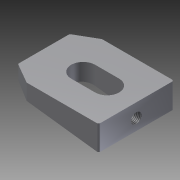
# Autodesk Inventor part: Wedge
Saved by Autodesk Inventor 2015 (Build 190159000, 159)
## iProperties
Shininess: 64.0
Angle Display Precision: 2
Document Length Units: 11272
Document Angle Units: 11279
Document Time Units: 11290
Document Mass Units: 11286
Document Length Units Precision: 3
Document Angle Units Precision: 2
Created: 2004-03-19
Part Number: Wedge
Document SubType Name: Modeling
Designer: bhandley
Material: Generic
Density: 1 g/cm^3
Appearance: Default
Density: 0.0
Volumn: 0.0
Area: 0.0
PropertySet Name: Model Information
Control State: 0
Master: False
Checked Out: False
Author: bhandley
Autodesk Inventor part; units mm, degrees
note: some values were not read from the file. Chosen so that the rebuilt part matches the saved one: direction of "Hole2".
ref_plane "YZ Plane" through (0, 0, 0) normal (1, 0, 0) x (0, 1, 0)
ref_plane "XZ Plane" through (0, 0, 0) normal (0, 1, 0) x (-1, 0, 0)
ref_plane "XY Plane" through (0, 0, 0) normal (0, 0, 1) x (1, 0, 0)
sketch "Sketch5" plane through (0, 0, 0) normal (0, 0, 1) x (1, 0, 0)
  line L0 (59.877, 38.0614) -> (231.327, 38.0614)
  line L1 (231.327, 38.0614) -> (231.327, -7.9761)
  line L2 (231.327, -7.9761) -> (59.877, -7.9761)
  line L3 (59.877, -7.9761) -> (59.877, 38.0614)
  dimension "d28" = 46.0375
  dimension "d29" = 171.45
  constraints: 8 end point, 2 parallel, 1 horizontal, 1 perpendicular
  measures "d28" distance of L0.end L1.end
  measures "d29" distance of L1.end L2.end
extrude "Extrusion4" add sketch "Sketch5" along normal blind 139.7
sketch "Sketch6" plane through (0, 0, 139.7) normal (0, 0, 1) x (1, 0, 0)
  line L0 (231.327, 38.0614) -> (231.327, -7.9761) projected
  line L1 (231.327, -7.9761) -> (59.877, -7.9761) projected
  line L2 (231.327, -7.9761) -> (-73.473, 30.1239)
  line L3 (-73.473, 30.1239) -> (-73.473, -7.9761)
  line L4 (59.877, -7.9761) -> (-73.473, -7.9761)
  dimension "d32" = 304.8
  dimension "d33" = 38.1
  constraints: 6 end point, 2 perpendicular
  measures "d32" distance between parallel lines of L0 L3
  measures "d33" distance of L2.end L3.end
extrude "Extrusion5" cut sketch "Sketch6" against normal through all
sketch "Sketch7" plane through (59.877, 38.0614, 0) normal (0, 1, 0) x (1, 0, 0)
  line L0 (0, -139.7) -> (171.45, -139.7) projected
  line L1 (0, 0) -> (0, -139.7) projected
  arc A0 (73.025, -47.625) -> (73.025, -92.075) centre (73.025, -69.85) ccw
  arc A1 (117.475, -92.075) -> (117.475, -47.625) centre (117.475, -69.85) ccw
  line L2 (73.025, -92.075) -> (117.475, -92.075)
  line L3 (73.025, -47.625) -> (117.475, -47.625)
  dimension "d36" = 69.85
  dimension "d37" = 22.225
  dimension "d38" = 73.025
  dimension "d39" = 44.45
  constraints: 4 end point, 4 point on circle, 4 tangent, 2 centre point, 1 equal radius, 1 parallel, 1 perpendicular
  measures "d36" distance from line of L0 A0.centre
  measures "d37" radius of A0
  measures "d38" distance from line of L1 A0.centre
  measures "d39" distance of A1.centre A0.centre
extrude "Extrusion6" cut sketch "Sketch7" against normal through all
sketch "Sketch8" plane through (59.877, 38.0614, 0) normal (0, 1, 0) x (1, 0, 0)
  line L0 (0, -139.7) -> (171.45, -139.7) projected
  line L1 (0, 0) -> (171.45, 0) projected
  line L2 (0, 0) -> (0, -139.7) projected
  line L3 (38.1, -139.7) -> (0, -117.703)
  line L4 (0, -21.997) -> (38.1, 0)
  dimension "d42" = 30
  dimension "d43" = 38.1
  dimension "d56" = 30
  constraints: 4 end point, 4 point on line, 1 equal length
  measures "d42" angle of L3 L0
  measures "d43" distance from line of L3.start L2
  measures "d56" angle of L4 L1
extrude "Extrusion7" cut sketch "Sketch8" against normal through all
sketch "Sketch9" plane through (231.327, 38.0614, 139.7) normal (1, 0, 0) x (0, 0, -1)
  line L0 (0, 0) -> (0, -46.0375) projected
  line L1 (139.7, 0) -> (0, 0) projected
  point P0 (69.85, -25.4)
  dimension "d46" = 69.85
  dimension "d47" = 25.4
  measures "d46" distance from line of point (69.85, -25.4) L0
  measures "d47" distance from line of point (69.85, -25.4) L1
hole "Hole2" at (231.327, 12.6614, 69.85) direction (-1, 0, 0) diameter 19.177 end up to surface thread size "7/8-9 UNC" class "1B" standard "ANSI Unified Screw Threads"
fillet "Fillet2" radius 3.175 6 edges at (97.977, 23.377, 139.7) (59.877, 25.7583, 117.703) (59.877, 25.7583, 21.997) (97.977, 23.377, 0) (231.327, 15.0427, 0) (231.327, 15.0427, 139.7)
body "Solid1"
